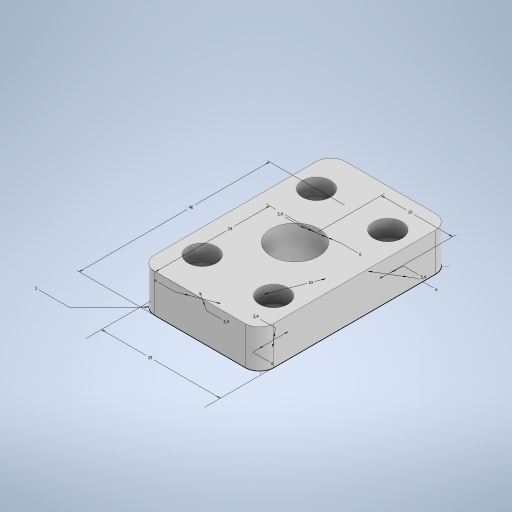
# Autodesk Inventor part: Adapterplatte_Focus
Saved by Autodesk Inventor 2024 (Build 280153000, 153)
## iProperties
Created: 2024-03-07
Part Number: Adapterplatte_Focus
Material: Generisch
Document SubType Name: Modeling
Designer: s1alknau
Density: 1 g/cm^3
Appearance: Vorgabe
Author: s1alknau
Autodesk Inventor part; units mm, degrees
ref_plane "YZ Plane" through (0, 0, 0) normal (1, 0, 0) x (0, 1, 0)
ref_plane "XZ Plane" through (0, 0, 0) normal (0, 1, 0) x (-1, 0, 0)
ref_plane "XY Plane" through (0, 0, 0) normal (0, 0, 1) x (1, 0, 0)
sketch "Skizze2" plane through (0, 0, 0) normal (0, 0, 1) x (1, 0, 0)
  line L0 (-9.5, -20) -> (9.5, -20)
  line L1 (12.5, -17) -> (12.5, 17)
  line L2 (9.5, 20) -> (-9.5, 20)
  line L3 (-12.5, 17) -> (-12.5, -17)
  line L4 (-12.5, -20) -> (12.5, 20) construction
  line L5 (12.5, -20) -> (-12.5, 20) construction
  circle A0 centre (0, 0) radius 5
  circle A1 centre (7.5, -12) radius 1.7
  circle A2 centre (-7.5, -12) radius 1.7
  circle A3 centre (7.5, 12) radius 1.7
  circle A4 centre (-7.5, 12) radius 1.7
  circle A5 centre (-7.5, 12) radius 3
  circle A6 centre (7.5, 12) radius 3
  circle A7 centre (7.5, -12) radius 3
  circle A8 centre (-7.5, -12) radius 3
  arc A9 (-12.5, -17) -> (-9.5, -20) centre (-9.5, -17) ccw
  arc A10 (9.5, -20) -> (12.5, -17) centre (9.5, -17) ccw
  arc A11 (12.5, 17) -> (9.5, 20) centre (9.5, 17) ccw
  arc A12 (-9.5, 20) -> (-12.5, 17) centre (-9.5, 17) ccw
  dimension "d0" = 40
  dimension "d1" = 25
  dimension "d9" = 10
  dimension "d11" = 3.4
  dimension "d12" = 3.4
  dimension "d13" = 3.4
  dimension "d14" = 3.4
  dimension "d15" = 15
  dimension "d16" = 24
  dimension "d17" = 6
  dimension "d18" = 6
  dimension "d19" = 6
  dimension "d20" = 6
  dimension "d21" = 3
  constraints: 13 centre point, 13 point on line, 12 end point, 8 point on circle, 8 tangent, 3 coincident, 3 equal radius, 2 midpoint, 2 parallel, 1 horizontal, 1 perpendicular
  measures "d0" distance between parallel lines of L2 L0
  measures "d1" distance between parallel lines of L1 L3
  measures "d9" diameter of A0
  measures "d11" diameter of A1
  measures "d12" diameter of A2
  measures "d13" diameter of A3
  measures "d14" diameter of A4
  measures "d15" distance of A3.centre A4.centre
  measures "d16" distance of A4.centre A2.centre
  measures "d17" diameter of A5
  measures "d18" diameter of A6
  measures "d19" diameter of A7
  measures "d20" diameter of A8
  measures "d21" radius of A9
extrude "Extrusion1" add sketch "Skizze2" along normal blind 8 contours A9 L3 A12 L2 A11 L1 A10 L0 | A0
extrude "Extrusion3" add sketch "Skizze2" along normal blind 4.6 contours A5 | A6 | A7 | A8
extrude "Extrusion4" cut sketch "Skizze2" along normal through all contours A0
